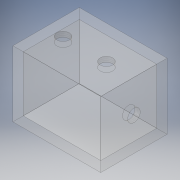
# Autodesk Inventor part: Reservoir
Saved by Autodesk Inventor 2018 (Build 220112000, 112)
## iProperties
Created: 2017-10-23
Part Number: Reservoir
Material: PMMA Plastic
Document SubType Name: Modeling
Designer: Gabriel Smolnycki
Density: 1.188 g/cm^3
Appearance: Polycarbonate - Clear
Author: Gabriel Smolnycki
Autodesk Inventor part; units mm, degrees
note: some values were not read from the file. Chosen so that the rebuilt part matches the saved one: direction of "Hole1"; direction of "Hole2".
ref_plane "YZ Plane" through (0, 0, 0) normal (1, 0, 0) x (0, 1, 0)
ref_plane "XZ Plane" through (0, 0, 0) normal (0, 1, 0) x (-1, 0, 0)
ref_plane "XY Plane" through (0, 0, 0) normal (0, 0, 1) x (1, 0, 0)
sketch "Sketch1" plane through (0, 0, 0) normal (0, 1, 0) x (-1, 0, 0)
  line L0 (-40.135, 30.32) -> (40.135, 30.32)
  line L1 (40.135, 30.32) -> (40.135, -30.32)
  line L2 (40.135, -30.32) -> (-40.135, -30.32)
  line L3 (-40.135, -30.32) -> (-40.135, 30.32)
  line L4 (-40.135, 30.32) -> (40.135, -30.32) construction
  line L5 (40.135, 30.32) -> (-40.135, -30.32) construction
  point P0 (0, 0)
  dimension "d0" = 80.27
  dimension "d1" = 60.64
  constraints: 12 end point, 2 midpoint, 2 parallel, 1 horizontal, 1 perpendicular
  measures "d0" distance of L1.end L2.end
  measures "d1" distance of L0.end L1.end
extrude "Extrusion1" add sketch "Sketch1" along normal blind 4.75
sketch "Sketch2" plane through (0, 4.75, 0) normal (0, 1, 0) x (1, 0, 0)
  line L0 (-40.135, -30.32) -> (40.135, -30.32) projected
  line L1 (40.135, -30.32) -> (40.135, 30.32) projected
  line L2 (-40.135, -30.32) -> (40.135, -30.32)
  line L3 (40.135, -30.32) -> (40.135, -25.57)
  line L4 (40.135, -25.57) -> (-40.135, -25.57)
  line L5 (-40.135, -25.57) -> (-40.135, -30.32)
  line L6 (-40.135, 30.32) -> (40.135, 30.32)
  line L7 (40.135, 30.32) -> (40.135, 25.57)
  line L8 (40.135, 25.57) -> (-40.135, 25.57)
  line L9 (-40.135, 25.57) -> (-40.135, 30.32)
  line L10 (-40.135, -25.57) -> (-35.385, -25.57)
  line L11 (-35.385, -25.57) -> (-35.385, 25.57)
  line L12 (-35.385, 25.57) -> (-40.135, 25.57)
  line L13 (-40.135, 25.57) -> (-40.135, -25.57)
  line L14 (40.135, 25.57) -> (35.385, 25.57)
  line L15 (35.385, 25.57) -> (35.385, -25.57)
  line L16 (35.385, -25.57) -> (40.135, -25.57)
  line L17 (40.135, -25.57) -> (40.135, 25.57)
  point P0 (0, 0)
  dimension "d4" = 4.75
  dimension "d5" = 4.75
  dimension "d6" = 4.75
  dimension "d7" = 4.75
  constraints: 32 end point, 8 parallel, 5 point on line, 4 horizontal, 4 perpendicular
  measures "d4" distance of L3.end L2.end
  measures "d5" distance of L1.end L7.end
  measures "d6" distance of L12.end L11.end
  measures "d7" distance of L16.end L15.end
extrude "Extrusion2" add sketch "Sketch2" along normal blind 50.72 contours L5 L4 L1 L0 | L13 L8 L11 L4 | L4 L15 L8 L1 | L9 L6 L1 L8
sketch "Sketch3" plane through (0, 55.47, 0) normal (0, 1, 0) x (1, 0, 0)
  line L0 (40.135, -30.32) -> (-40.135, -30.32) projected
  line L1 (-40.135, -30.32) -> (-40.135, 30.32) projected
  line L2 (-40.135, 30.32) -> (40.135, 30.32) projected
  line L3 (40.135, 30.32) -> (40.135, -30.32) projected
  point P0 (0, 0)
extrude "Extrusion3" add sketch "Sketch3" along normal blind 4.75
sketch "Sketch4" plane through (40.135, 0, 30.32) normal (1, 0, 0) x (0, 0, -1)
  line L0 (0, 60.22) -> (60.64, 60.22) projected
  line L1 (0, 0) -> (0, 60.22) projected
  line L2 (60.64, 0) -> (60.64, 60.22) projected
  line L3 (60.64, 0) -> (0, 0) projected
  point P0 (30.32, 0)
  point P1 (30.32, 30.11)
hole "Hole1" at (40.135, 30.11, 0) direction (-1, 0, 0) diameter 11.4554 end up to surface
sketch "Sketch5" plane through (0, 60.22, 0) normal (0, 1, 0) x (1, 0, 0)
  line L0 (-40.135, -30.32) -> (40.135, -30.32) projected
  line L1 (40.135, -30.32) -> (40.135, 30.32) projected
  line L2 (40.135, 30.32) -> (-40.135, 30.32) projected
  line L3 (-40.135, 30.32) -> (-40.135, -30.32) projected
  point P0 (0, 0)
  point P1 (-24.635, 0)
  point P2 (15.015, 0)
  dimension "d19" = 15.5
  dimension "d20" = 25.12
  measures "d19" distance from line of L3 point (-24.635, 0)
  measures "d20" distance from line of L1 point (15.015, 0)
hole "Hole2" at (-24.635, 60.22, 0) at (15.015, 60.22, 0) direction (0, -1, 0) diameter 11.4554 end up to surface
body "Solid1"
